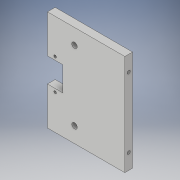
# Autodesk Inventor part: left side
Saved by Autodesk Inventor 2017 (Build 210142000, 142)
## iProperties
Created: 2016-07-21
Part Number: left side
Material: Generic
Document SubType Name: Modeling
Designer: Darien Morrow
Density: 1 g/cm^3
Appearance: Default
Author: Darien Morrow
Autodesk Inventor part; units mm, degrees
ref_plane "YZ Plane" through (0, 0, 0) normal (1, 0, 0) x (0, 1, 0)
ref_plane "XZ Plane" through (0, 0, 0) normal (0, 1, 0) x (-1, 0, 0)
ref_plane "XY Plane" through (0, 0, 0) normal (0, 0, 1) x (1, 0, 0)
sketch "Sketch1" plane through (0, 0, 0) normal (0, 0, 1) x (1, 0, 0)
  line L0 (-31.75, -41.275) -> (31.75, -41.275)
  line L1 (31.75, -41.275) -> (31.75, 41.275)
  line L2 (31.75, 41.275) -> (-31.75, 41.275)
  line L3 (-31.75, 41.275) -> (-31.75, -41.275)
  line L4 (-31.75, -41.275) -> (31.75, 41.275) construction
  line L5 (31.75, -41.275) -> (-31.75, 41.275) construction
  point P0 (0, 0)
  dimension "d0" = 63.5
  dimension "d1" = 82.55
  constraints: 12 end point, 2 midpoint, 2 parallel, 1 horizontal, 1 perpendicular
  measures "d0" distance of L2.end L1.end
  measures "d1" distance of L1.end L0.end
extrude "Extrusion1" add sketch "Sketch1" along normal blind 6.35
sketch "Sketch2" plane through (0, 0, 0) normal (0, 0, -1) x (-1, 0, 0)
  line L0 (44.45, -10) -> (19.05, -10)
  line L1 (19.05, -10) -> (19.05, 10)
  line L2 (19.05, 10) -> (44.45, 10)
  line L3 (44.45, 10) -> (44.45, -10)
  line L4 (31.75, 41.275) -> (31.75, -41.275) projected
  line L5 (44.45, -10) -> (19.05, 10) construction
  line L6 (19.05, -10) -> (44.45, 10) construction
  point P0 (0, 0)
  point P1 (31.75, 0)
  dimension "d4" = 25.4
  dimension "d5" = 20
  constraints: 12 end point, 3 midpoint, 2 parallel, 1 horizontal, 1 perpendicular
  measures "d4" distance of L1.end L2.end
  measures "d5" distance between parallel lines of L0 L2
extrude "Extrusion2" cut sketch "Sketch2" against normal blind 6.35
sketch "Sketch3" plane through (0, 0, 0) normal (0, 0, -1) x (-1, 0, 0)
  line L0 (25.4, 12.7) -> (25.4, -12.7)
  line L1 (31.75, 41.275) -> (31.75, 10) projected
  point P0 (0, 0)
  dimension "d8" = 12.7
  dimension "d9" = 25.4
  dimension "d10" = 6.35
  constraints: 2 coincident, 2 end point, 1 vertical
  measures "d8" vertical distance of point (0, 0) L0.start
  measures "d9" distance of L0.end L0.start
  measures "d10" distance between parallel lines of L1 L0
hole "Hole1" at (-25.4, 12.7, 0) at (-25.4, -12.7, 0) direction (0, 0, 1) diameter 2.159 end through all
sketch "Sketch4" plane through (0, 0, 0) normal (0, 0, -1) x (-1, 0, 0)
  line L0 (9.525, 28.575) -> (9.525, -28.575)
  line L1 (-31.75, 41.275) -> (31.75, 41.275) projected
  line L2 (19.05, -10) -> (19.05, 10) projected
  point P0 (0, 0)
  dimension "d18" = 57.15
  dimension "d19" = 12.7
  dimension "d20" = 9.525
  constraints: 2 coincident, 2 end point, 1 vertical
  measures "d18" distance of L0.start L0.end
  measures "d19" distance from line of L0.start L1
  measures "d20" distance between parallel lines of L2 L0
hole "Hole2" at (-9.525, 28.575, 0) at (-9.525, -28.575, 0) direction (0, 0, 1) diameter 4.4958 depth 12.2936 tip angle 118 counterbore diameter 7.9502 counterbore depth 2.54 clearance for "Socket Head Cap Screw" size "#8" standard "Ansi Unified Screw Threads"
sketch "Sketch5" plane through (31.75, -41.275, 0) normal (1, 0, 0) x (0, 0, -1)
  line L0 (-3.175, 69.85) -> (-3.175, 12.7)
  line L1 (-6.35, 0) -> (-6.35, 82.55) projected
  line L2 (0, 82.55) -> (-6.35, 82.55) projected
  point P0 (0, 41.275)
  dimension "d28" = 57.15
  dimension "d29" = 12.7
  dimension "d30" = 3.175
  constraints: 2 coincident, 2 end point, 1 parallel
  measures "d28" distance of L0.end L0.start
  measures "d29" distance from line of L0.start L2
  measures "d30" distance between parallel lines of L0 L1
hole "Hole3" at (31.75, 28.575, 3.175) at (31.75, -28.575, 3.175) direction (-1, 0, 0) diameter 2.6416 depth 10.9728 tip angle 118 thread size "6-32 UNC" class "2B" standard "ANSI Unified Screw Threads"
body "Solid1"
